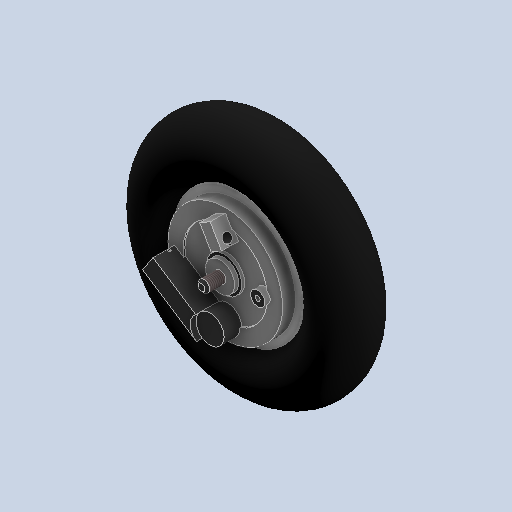
# Autodesk Inventor part: FreeBackWheel
Saved by Autodesk Inventor 2022.2 (Build 262287000, 287)
## iProperties
Created: 2022-03-30
Part Number: FreeBackWheel
Material: Rubber
Document SubType Name: Modeling
Designer: Finn Oriwohl
Density: 0.93 g/cm^3
Appearance: Rubber - Black
Mass: 1197.34 g
Surface Area: 982.206 cm^2
Volume: 1287.46 cm^3
Author: Finn Oriwohl
Autodesk Inventor part; units mm, degrees
ref_plane "YZ Plane" through (0, 0, 0) normal (1, 0, 0) x (0, 1, 0)
ref_plane "XZ Plane" through (0, 0, 0) normal (0, 1, 0) x (-1, 0, 0)
ref_plane "XY Plane" through (0, 0, 0) normal (0, 0, 1) x (1, 0, 0)
sketch "Sketch2" plane through (0, 0, 0) normal (1, 0, 0) x (0, 1, 0)
  line L0 (17.5, 10.75) -> (-17.5, 10.75)
  line L1 (-17.5, 10.75) -> (-17.5, -28.75)
  line L2 (-17.5, -28.75) -> (17.5, -28.75)
  line L3 (17.5, -28.75) -> (17.5, 10.75)
  line L4 (17.5, 10.75) -> (-17.5, -28.75) construction
  line L5 (-17.5, 10.75) -> (17.5, -28.75) construction
  line L6 (-55, -9.75) -> (55, -9.75)
  line L7 (55, -9.75) -> (55, -15.4999)
  line L8 (55, -15.4999) -> (-55, -15.4999)
  line L9 (-55, -15.4999) -> (-55, -9.75)
  line L10 (-55, -9.75) -> (55, -15.4999) construction
  line L11 (55, -9.75) -> (-55, -15.4999) construction
  line L12 (46, -9.75) -> (46, -15.4999)
  line L13 (0, 65.9057) -> (0, -65.9057)
  circle A0 centre (75.7124, 0) radius 25
  line L14 (0, 0) -> (82.4805, 0) construction
  line L15 (-55, 9.75) -> (55, 9.75)
  line L16 (55, 9.75) -> (55, 15.4999)
  line L17 (55, 15.4999) -> (-55, 15.4999)
  line L18 (-55, 15.4999) -> (-55, 9.75)
  line L19 (46, 9.75) -> (46, 15.4999)
  line L20 (0, 24.9999) -> (49, 24.9999)
  line L21 (49, 24.9999) -> (49, 15.4999)
  line L22 (0, 30.9999) -> (12.5, 30.9999)
  line L23 (12.5, 30.9999) -> (12.5, 24.9999)
  line L24 (0, -28.75) -> (5, -28.75)
  line L25 (5, -28.75) -> (5, -46.25)
  line L26 (5, -46.25) -> (0, -46.25)
  line L27 (0, -46.25) -> (0, -28.75)
  line L28 (0, 30.9999) -> (5, 30.9999)
  line L29 (5, 30.9999) -> (5, 46.7999)
  line L30 (5, 46.7999) -> (0, 46.7999)
  line L31 (0, 46.7999) -> (0, 30.9999)
  point P0 (0, -9)
  point P1 (0, -9)
  point P2 (0, -12.625)
  point P3 (0, -12.625)
  point P4 (0, -12.625)
  point P5 (0, -9)
  point P6 (55, -13.9999)
  point P7 (0, 12.625)
  point P8 (55, 13.9999)
  point P9 (55, 13.9999)
  point P10 (0, -30)
  point P11 (17.5, -15.4999)
  point P12 (0, -46.25)
  point P13 (5, -28.75)
  point P14 (0, 46.7999)
  point P15 (5, 30.9999)
  point P16 (99.7681, -6.8058)
  point P17 (0, 10.75)
  point P18 (17.5, -9.75)
  dimension "d0" = 35
  dimension "d1" = 39.5
  dimension "d2" = 9
  dimension "d3" = 110
  dimension "d7" = 9
  dimension "d12" = 49
  dimension "d13" = 9.5
  dimension "d14" = 12.5
  dimension "d15" = 6
  dimension "d42" = 5
  dimension "d43" = 17.5
  dimension "d44" = 5
  dimension "d45" = 15.8
  dimension "d53" = 100
  dimension "d74" = 19
  dimension "d75" = 50
  dimension "d76" = 1.5
  constraints: 64 end point, 14 point on line, 10 midpoint, 8 parallel, 8 symmetric about line, 7 horizontal, 5 perpendicular, 3 vertical, 2 coincident, 2 point on circle, 1 centre point
  measures "d0" distance of L2.end L1.end
  measures "d1" distance of L1.end L0.end
  measures "d2" distance of point (0, -9) point (0, 0)
  measures "d3" distance of L7.end L8.end
  measures "d7" distance between parallel lines of L7 L12
  measures "d12" distance of L20.start L20.end
  measures "d13" distance between parallel lines of L17 L20
  measures "d14" distance of L22.start L22.end
  measures "d15" distance between parallel lines of L20 L22
  measures "d42" distance of L25.end L26.end
  measures "d43" distance of L24.end L25.end
  measures "d44" distance of L30.end L29.end
  measures "d45" distance of L29.end L28.end
  measures "d53" distance of point (0, 0) A0.end
  measures "d74" distance between parallel lines of L6 L2
  measures "d75" diameter of A0
  measures "d76" distance from line of L8 A0.start
revolve "Revolution1" add sketch "Sketch2" angle 360 about axis through (0, 0, 65.9057) along (0, 0, -1) contours L3 L15 L13 L0 | L0 L13 L17 L19 L15 L3 | L15 A0 L6 L3 | L3 L6 L13 L15 | L13 L20 L21 L17 | L3 L8 L13 L6 | L19 L17 L16 A0 L15 | L13 L22 L23 L20 | L3 L2 L13 L8 | L6 A0 L7 L8 L12 | L15 L16 A0 L7 L6 | A0 L16 L15 | L13 L30 L29 L22 | L6 L7 A0 | L2 L25 L26 L13
sketch "Sketch4" plane through (0, 0, 24.9999) normal (0, 0, 1) x (1, 0, 0)
  circle A0 centre (32.15, 0) radius 6.15
  circle A1 centre (32.15, 0) radius 2.15
  circle A2 centre (0, 0) radius 49 projected
  circle A3 centre (0, 0) radius 49 projected
  line L0 (26, 14.6294) -> (26, -8.2066)
  circle A4 centre (0, 0) radius 36
  circle A5 centre (0, 0) radius 15
  line L1 (-8.8861, 39.8) -> (0.1206, 45)
  line L2 (0.1206, 45) -> (9.8706, 28.1125)
  line L3 (9.8706, 28.1125) -> (0.8639, 22.9125)
  line L4 (0.8639, 22.9125) -> (-8.8861, 39.8)
  line L5 (-8.8861, 39.8) -> (9.8706, 28.1125) construction
  line L6 (0.1206, 45) -> (0.8639, 22.9125) construction
  line L7 (0, 0) -> (49, 0) construction
  circle A6 centre (0.4923, -33.9563) radius 12
  line L8 (0.5569, -29.2189) -> (-43.347, -0.503)
  line L9 (-43.347, -0.503) -> (-52.105, -13.8932)
  line L10 (-52.105, -13.8932) -> (-6.0762, -43.9989)
  line L11 (-4.0111, 31.3563) -> (-50.7764, 4.3563) construction
  point P0 (0, 0)
  point P1 (0.4923, 33.9563)
  point P2 (5.5667, 35.567)
  point P3 (35.6423, 5.0622)
  point P4 (35.6423, -5.0622)
  point P5 (-6.3647, 35.4329)
  point P6 (0.4923, 33.9563)
  point P7 (-6.7865, -24.4159)
  point P8 (-48.9, 3.1289)
  point P9 (-45.4855, -18.2228)
  point P10 (-48.3238, -8.1121)
  dimension "d55" = 24
  dimension "d24" = 12.3
  dimension "d25" = 4
  dimension "d26" = 23
  dimension "d29" = 72
  dimension "d30" = 30
  dimension "d31" = 10.4
  dimension "d32" = 19.5
  dimension "d33" = 60
  dimension "d34" = 98
  dimension "d35" = 45
  dimension "d54" = 46.4246
  dimension "d56" = 16
  dimension "d57" = 54
  dimension "d62" = 55
  constraints: 24 end point, 4 centre point, 4 midpoint, 3 coincident, 3 parallel, 3 perpendicular, 2 point on line, 1 horizontal, 1 horizontal alignment, 1 symmetric about line, 1 tangent, 1 vertical, 5 other
  measures "d24" diameter of A0
  measures "d25" radial gap between concentric circles of A0 A1
  measures "d26" distance from line of L7.end L0
  measures "d29" diameter of A4
  measures "d30" diameter of A5
  measures "d31" distance of L2.end L3.end
  measures "d32" distance of L1.end L2.end
  measures "d33" angle of L0 L3
  measures "d34" diameter of A2
  measures "d35" vertical distance of A2.centre L1.end
  measures "d54" distance of A0.centre point (0.492, 33.956)
  measures "d56" distance of L8.end L9.end
  measures "d57" distance of L11.start L11.end
  measures "d62" distance from line of point (0.492, -33.956) L9
extrude "Extrusion1" add sketch "Sketch4" along normal blind 6 contours A0 A4 | A4 A0
extrude "Extrusion2" add sketch "Sketch4" along normal blind 1.5 contours A0 A4 L2 L1 L4 L8 L9 A2 L10 A6 | A6 A4 | A6 L10 A2 L9 L8 A4 picked at (0.1047, -39.1419)
extrude "Extrusion3" add sketch "Sketch4" along normal blind 2.5 contours A5
extrude "Extrusion4" add sketch "Sketch4" along normal blind 14.5 contours L2 L3 L4 A4 | A4 L4 L1 L2
sketch "Sketch3" plane through (0, 0, 30.9999) normal (0, 0, 1) x (1, 0, 0)
  point P0 (0, 0)
  point P1 (0, 0)
  constraints: 1 coincident
hole "Hole1" [suppressed]
chamfer "Chamfer1" distance 2 angle 45 2 edges at (0, -5, 46.7999) (0, -5, -46.25)
thread "Thread1" size "M10x1.5" class "6g" standard "ANSI Metric M Profile" length 14 offset 3.5
thread "Thread2" size "M10x1.5" class "6g" standard "ANSI Metric M Profile" full length
extrude "Extrusion5" add sketch "Sketch4" along normal blind 15 contours A6 A4 | A4 A6
extrude "Extrusion6" add sketch "Sketch4" along normal blind 20 contours A6 L10 A2 L9 L8 A4 | A4 L8 A6 | L10 L9 A2
sketch "Sketch5" plane through (9.8706, 28.1125, 39.4999) normal (0.866, 0.5, 0) x (0, 0, -1)
  line L0 (13, 19.5) -> (13, 8.6077) projected
  line L1 (13, 19.5) -> (0, 19.5) projected
  line L2 (0, 0) -> (0, 19.5) projected
  line L3 (14.5, 0) -> (0, 0) projected
  line L4 (14.5, 8.6077) -> (14.5, 0) projected
  line L5 (14.5, 8.6077) -> (13, 8.6077) projected
  circle A0 centre (7.5, 5.5) radius 4
  line L6 (3.5, 17.7174) -> (3.5, 4.9566) construction
  line L7 (3.5, 9.5) -> (10.4741, 9.5) construction
  line L8 (14.5, 0) -> (0, 0) projected
  line L9 (6.5, 0) -> (6.5, 5.5)
  line L10 (8.5, 5.5) -> (8.5, 0)
  line L11 (6.5, 5.5) -> (8.5, 5.5) construction
  point P0 (39.4999, -19.4108)
  point P1 (8.5, 2.75)
  point P2 (6.5, 2.75)
  point P3 (6.5, 1.627)
  point P4 (6.5, 0)
  point P5 (8.5, 1.627)
  dimension "d63" = 8
  dimension "d64" = 3.5
  dimension "d65" = 10
  dimension "d66" = 2
  constraints: 10 end point, 3 midpoint, 3 point on line, 2 perpendicular, 2 tangent, 1 centre point, 1 coincident, 1 horizontal, 1 parallel, 1 vertical
  measures "d63" diameter of A0
  measures "d64" distance between parallel lines of L2 L6
  measures "d65" distance between parallel lines of L1 L7
  measures "d66" distance of point (8.5, 2.75) point (6.5, 2.75)
extrude "Extrusion7" cut sketch "Sketch5" against normal up to surface (10.4 mm away) contours L9 A0 L10 L3 | A0
extrude "Extrusion8" cut sketch "Sketch5" against normal through all contours L9 A0 L10 L3
thread "Thread3" size "M4.5x0.75" class "6H" standard "ANSI Metric M Profile" full length
equation "\"d42\" = d44"
body "Solid1"
